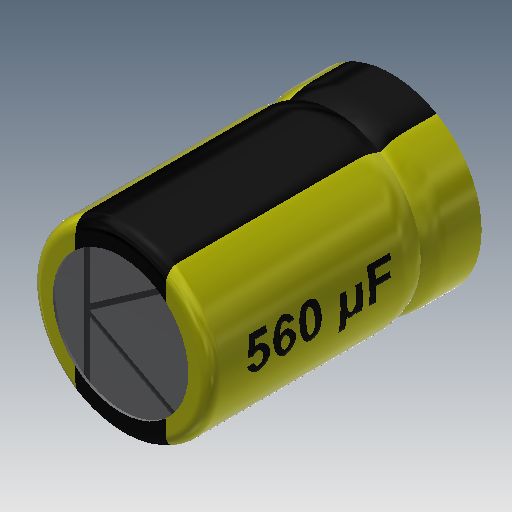
# Autodesk Inventor part: config - capasitor 560 μF
Saved by Autodesk Inventor 2020 (Build 240152000, 152)
## iProperties
Created: 2005-12-06
Part Number: config - capasitor 560 μF
Document SubType Name: Modeling
Designer: Simon.Ng@autodesk.com
Stock Number: config - capasitor 560 μF
Density: 1 g/cm^3
Material: Generic
Mass: 0.595409 g
Surface Area: 4.0268 cm^2
Volume: 0.595409 cm^3
Appearance: Smooth - Yellow
Company: Autodesk Asia Pte. Ltd.
Title: PC Demo
Author: Simon.Ng@autodesk.com
Autodesk Inventor part; units mm, degrees
ref_plane "YZ Plane" through (0, 0, 0) normal (1, 0, 0) x (0, 1, 0)
ref_plane "XZ Plane" through (0, 0, 0) normal (0, 1, 0) x (-1, 0, 0)
sketch "Sketch1" plane through (0, 0, 0) normal (0, 0, 1) x (1, 0, 0)
  line L0 (0, 6.4) -> (0, -4.8) construction
  line L1 (-4.8, 0) -> (6.4, 0) construction
  circle A0 centre (0, 0) radius 4
  dimension "d0" = 8
  constraints: 2 point on line, 1 centre point
  measures "d0" diameter of A0
extrude "Extrusion1" add sketch "Sketch1" along normal blind 12
sketch "Sketch6" plane through (0, 0, 0) normal (1, 0, 0) x (0, 1, 0)
  line L0 (0, 15.6) -> (0, -1.2) projected
  line L1 (4, 0) -> (4, 12) projected
  line L2 (4, 3.5) -> (4, 1.5)
  line L3 (4, 2.5) -> (3.8, 2.5) construction
  line L4 (-4, 0) -> (4, 0) construction
  arc A0 (3.8, 2.5) -> (4, 3.5) centre (1.4, 3.5) ccw
  arc A1 (4, 1.5) -> (3.8, 2.5) centre (1.4, 1.5) ccw
  point P0 (0, 0)
  dimension "d16" = 2
  dimension "d17" = 2.5
  dimension "d18" = 0.2
  constraints: 4 end point, 4 point on circle, 2 centre point, 2 point on line, 2 tangent, 1 collinear, 1 horizontal, 1 midpoint
  measures "d16" distance of L2.start L2.end
  measures "d17" distance between parallel lines of L4 L3
  measures "d18" distance of L3.start L3.end
revolve "Revolution1" cut sketch "Sketch6" angle 360 about axis through (0, 0, 0) along (0, 0, -1)
sketch "Sketch2" plane through (0, 0, 12) normal (0, 0, 1) x (1, 0, 0)
  circle A0 centre (0, 0) radius 4 projected
  circle A1 centre (0, 0) radius 3
  dimension "d3" = 1
  constraints: 1 centre point, 1 coincident
  measures "d3" radial gap between concentric circles of A1 A0
extrude "Extrusion2" cut sketch "Sketch2" against normal blind 0.1 contours A1
sketch "Sketch3" plane through (0, 0, 11.9) normal (0, 0, 1) x (1, 0, 0)
  line L0 (-1.7345, 2.8958) -> (-1.4712, 2.8958)
  line L1 (-1.4712, 2.8958) -> (-1.4712, -3.0531)
  line L2 (-1.4712, -3.0531) -> (-1.7345, -3.0531)
  line L3 (-1.7345, -3.0531) -> (-1.7345, 2.8958)
  line L4 (-1.4712, 0.1227) -> (-1.5962, 0.3017)
  line L5 (-1.5962, 0.3017) -> (1.7965, 2.6719)
  line L6 (1.7965, 2.6719) -> (1.9215, 2.493)
  line L7 (1.9215, 2.493) -> (-1.4712, 0.1227)
  line L8 (-1.4712, 0.1227) -> (-1.5776, -0.0787)
  line L9 (-1.5776, -0.0787) -> (2.3639, -2.1618)
  line L10 (2.3639, -2.1618) -> (2.4704, -1.9604)
  line L11 (2.4704, -1.9604) -> (-1.4712, 0.1227)
  constraints: 24 end point, 6 parallel, 3 perpendicular, 1 horizontal, 1 point on line
extrude "Extrusion3" cut sketch "Sketch3" against normal blind 0.05
fillet "Fillet1" radius 0.5 1 edges at (-4, 0, 12)
sketch "Sketch5" plane through (0, 0, 12) normal (0, 0, 1) x (1, 0, 0)
  circle A0 centre (0, 0) radius 3 projected
  circle A1 centre (0, 0) radius 4 projected
  line L0 (2, -2.2361) -> (2, -5)
  line L1 (2, -5) -> (-2, -5)
  line L2 (-2, -5) -> (-2, -2.2361)
  line L3 (0, -4.8) -> (0, 6.4) projected
  point P0 (0, -4)
  point P1 (0, -4)
  dimension "d12" = 1
  dimension "d13" = 4
  constraints: 6 end point, 2 point on circle, 1 coincident, 1 parallel, 1 point on line, 1 vertical alignment, 2 other
  measures "d12" distance from line of L1 point (0, -4)
  measures "d13" distance of L0.end L1.end
split_face "Split1"
ref_plane "Work Plane1" through (10, 0, 0) normal (1, 0, 0) x (0, 1, 0)
sketch "Sketch4" plane through (10, 0, 0) normal (1, 0, 0) x (0, 0, -1)
  line L0 (-10.4753, 1.0434) -> (5.133, 1.0434) construction
  line L1 (5.133, 1.0434) -> (5.133, -2.7958) construction
  line L2 (5.133, -2.7958) -> (-10.4753, -2.7958) construction
  line L3 (-10.4753, -2.7958) -> (-10.4753, 1.0434) construction
  line L4 (-10.3827, -0.077) -> (-10.0957, -0.0473)
  spline S0 degree 3 poles (-10.0957, -0.0473) (-10.0831, -0.1445) (-9.9631, -0.2577) (-9.8842, -0.2577) knots 0 0 0 0 1 1 1 1
  spline S1 degree 3 poles (-9.8842, -0.2577) (-9.7939, -0.2577) (-9.6692, -0.1113) (-9.6692, 0.0373) knots 0 0 0 0 1 1 1 1
  spline S2 degree 3 poles (-9.6692, 0.0373) (-9.6692, 0.1756) (-9.7939, 0.314) (-9.8933, 0.314) knots 0 0 0 0 1 1 1 1
  spline S3 degree 2 poles (-9.8933, 0.314) (-10.0168, 0.314) (-10.1151, 0.2042) knots 0 0 0 1 1 1
  line L5 (-10.1151, 0.2042) -> (-10.3484, 0.2385)
  line L6 (-10.3484, 0.2385) -> (-10.2009, 1.0182)
  line L7 (-10.2009, 1.0182) -> (-9.4394, 1.0182)
  line L8 (-9.4394, 1.0182) -> (-9.4394, 0.7496)
  line L9 (-9.4394, 0.7496) -> (-9.9825, 0.7496)
  line L10 (-9.9825, 0.7496) -> (-10.0282, 0.4946)
  spline S4 degree 2 poles (-10.0282, 0.4946) (-9.9322, 0.5426) (-9.8316, 0.5426) knots 0 0 0 1 1 1
  spline S5 degree 3 poles (-9.8316, 0.5426) (-9.6395, 0.5426) (-9.3731, 0.2637) (-9.3731, 0.0419) knots 0 0 0 0 1 1 1 1
  spline S6 degree 2 poles (-9.3731, 0.0419) (-9.3731, -0.1434) (-9.4806, -0.2886) knots 0 0 0 1 1 1
  spline S7 degree 2 poles (-9.4806, -0.2886) (-9.6269, -0.4875) (-9.8876, -0.4875) knots 0 0 0 1 1 1
  spline S8 degree 3 poles (-9.8876, -0.4875) (-10.0945, -0.4875) (-10.3575, -0.2645) (-10.3827, -0.077) knots 0 0 0 0 1 1 1 1
  line L11 (-8.247, 0.6707) -> (-8.5248, 0.6398)
  spline S9 degree 3 poles (-8.5248, 0.6398) (-8.5351, 0.7255) (-8.6208, 0.8067) (-8.6894, 0.8067) knots 0 0 0 0 1 1 1 1
  spline S10 degree 3 poles (-8.6894, 0.8067) (-8.7809, 0.8067) (-8.9067, 0.6432) (-8.9227, 0.3848) knots 0 0 0 0 1 1 1 1
  spline S11 degree 2 poles (-8.9227, 0.3848) (-8.8163, 0.5117) (-8.6563, 0.5117) knots 0 0 0 1 1 1
  spline S12 degree 3 poles (-8.6563, 0.5117) (-8.4768, 0.5117) (-8.2195, 0.2374) (-8.2195, 0.0213) knots 0 0 0 0 1 1 1 1
  spline S13 degree 3 poles (-8.2195, 0.0213) (-8.2195, -0.2097) (-8.4894, -0.4875) (-8.7009, -0.4875) knots 0 0 0 0 1 1 1 1
  spline S14 degree 3 poles (-8.7009, -0.4875) (-8.9284, -0.4875) (-9.2211, -0.1342) (-9.2211, 0.2671) knots 0 0 0 0 1 1 1 1
  spline S15 degree 3 poles (-9.2211, 0.2671) (-9.2211, 0.6798) (-8.9158, 1.0434) (-8.6723, 1.0434) knots 0 0 0 0 1 1 1 1
  spline S16 degree 3 poles (-8.6723, 1.0434) (-8.5019, 1.0434) (-8.2779, 0.8524) (-8.247, 0.6707) knots 0 0 0 0 1 1 1 1
  spline S17 degree 3 poles (-8.8987, 0.0441) (-8.8987, -0.0965) (-8.7695, -0.2485) (-8.6872, -0.2485) knots 0 0 0 0 1 1 1 1
  spline S18 degree 3 poles (-8.6872, -0.2485) (-8.6071, -0.2485) (-8.5008, -0.1239) (-8.5008, 0.0178) knots 0 0 0 0 1 1 1 1
  spline S19 degree 3 poles (-8.5008, 0.0178) (-8.5008, 0.1642) (-8.6151, 0.3002) (-8.7009, 0.3002) knots 0 0 0 0 1 1 1 1
  spline S20 degree 3 poles (-8.7009, 0.3002) (-8.7843, 0.3002) (-8.8987, 0.1699) (-8.8987, 0.0441) knots 0 0 0 0 1 1 1 1
  spline S21 degree 2 poles (-7.5702, 1.0434) (-7.3518, 1.0434) (-7.2295, 0.8879) knots 0 0 0 1 1 1
  spline S22 degree 2 poles (-7.2295, 0.8879) (-7.0831, 0.7038) (-7.0831, 0.2774) knots 0 0 0 1 1 1
  spline S23 degree 2 poles (-7.0831, 0.2774) (-7.0831, -0.1479) (-7.2306, -0.3343) knots 0 0 0 1 1 1
  spline S24 degree 2 poles (-7.2306, -0.3343) (-7.3518, -0.4875) (-7.5702, -0.4875) knots 0 0 0 1 1 1
  spline S25 degree 3 poles (-7.5702, -0.4875) (-7.7897, -0.4875) (-8.0572, -0.1514) (-8.0572, 0.2808) knots 0 0 0 0 1 1 1 1
  spline S26 degree 2 poles (-8.0572, 0.2808) (-8.0572, 0.7038) (-7.9097, 0.8902) knots 0 0 0 1 1 1
  spline S27 degree 2 poles (-7.9097, 0.8902) (-7.7885, 1.0434) (-7.5702, 1.0434) knots 0 0 0 1 1 1
  spline S28 degree 3 poles (-7.5702, 0.8044) (-7.6227, 0.8044) (-7.7039, 0.7381) (-7.7268, 0.6524) knots 0 0 0 0 1 1 1 1
  spline S29 degree 2 poles (-7.7268, 0.6524) (-7.7565, 0.5415) (-7.7565, 0.2774) knots 0 0 0 1 1 1
  spline S30 degree 4 poles (-7.7565, 0.2774) (-7.7565, 0.0144) (-7.7028, -0.1834) (-7.6227, -0.2485) (-7.5702, -0.2485) knots 0 0 0 0 0 1 1 1 1 1
  spline S31 degree 3 poles (-7.5702, -0.2485) (-7.5176, -0.2485) (-7.4364, -0.1822) (-7.4135, -0.0965) knots 0 0 0 0 1 1 1 1
  spline S32 degree 2 poles (-7.4135, -0.0965) (-7.3838, 0.0144) (-7.3838, 0.2774) knots 0 0 0 1 1 1
  spline S33 degree 4 poles (-7.3838, 0.2774) (-7.3838, 0.5415) (-7.4375, 0.7381) (-7.5176, 0.8044) (-7.5702, 0.8044) knots 0 0 0 0 0 1 1 1 1 1
  line L12 (-6.2508, 0.6249) -> (-5.9627, 0.6249)
  line L13 (-5.9627, 0.6249) -> (-5.9627, 0.131)
  spline S34 degree 4 poles (-5.9627, 0.131) (-5.9627, -0.0073) (-5.9341, -0.1628) (-5.8335, -0.2588) (-5.7626, -0.2588) knots 0 0 0 0 0 1 1 1 1 1
  spline S35 degree 4 poles (-5.7626, -0.2588) (-5.6894, -0.2588) (-5.5831, -0.1582) (-5.5522, -0.0153) (-5.5522, 0.1276) knots 0 0 0 0 0 1 1 1 1 1
  line L14 (-5.5522, 0.1276) -> (-5.5522, 0.6249)
  line L15 (-5.5522, 0.6249) -> (-5.2641, 0.6249)
  line L16 (-5.2641, 0.6249) -> (-5.2641, -0.4623)
  line L17 (-5.2641, -0.4623) -> (-5.5294, -0.4623)
  line L18 (-5.5294, -0.4623) -> (-5.5294, -0.3309)
  spline S36 degree 2 poles (-5.5294, -0.3309) (-5.6094, -0.4863) (-5.7477, -0.4863) knots 0 0 0 1 1 1
  spline S37 degree 2 poles (-5.7477, -0.4863) (-5.8941, -0.4863) (-5.9627, -0.3309) knots 0 0 0 1 1 1
  line L19 (-5.9627, -0.3309) -> (-5.9627, -0.8762)
  line L20 (-5.9627, -0.8762) -> (-6.2508, -0.8762)
  line L21 (-6.2508, -0.8762) -> (-6.2508, 0.6249)
  line L22 (-4.9634, -0.4623) -> (-4.9634, 1.0377)
  line L23 (-4.9634, 1.0377) -> (-3.9333, 1.0377)
  line L24 (-3.9333, 1.0377) -> (-3.9333, 0.7839)
  line L25 (-3.9333, 0.7839) -> (-4.6605, 0.7839)
  line L26 (-4.6605, 0.7839) -> (-4.6605, 0.4294)
  line L27 (-4.6605, 0.4294) -> (-4.0328, 0.4294)
  line L28 (-4.0328, 0.4294) -> (-4.0328, 0.1756)
  line L29 (-4.0328, 0.1756) -> (-4.6605, 0.1756)
  line L30 (-4.6605, 0.1756) -> (-4.6605, -0.4623)
  line L31 (-4.6605, -0.4623) -> (-4.9634, -0.4623)
  constraints: 2 other
emboss "Emboss1" sketch "Sketch4" operation cut depth 0.05 direction (1, 0, 0) wrap yes faces at (-0.4906, 3.9698, 6.1667) (3.9468, -0.6414, 11.5374) (-0.4906, 3.9698, 1)
body "Solid1"
